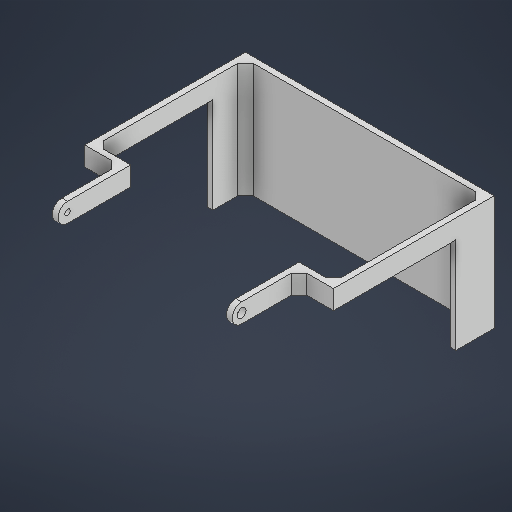
# Autodesk Inventor part: Arm
Saved by Autodesk Inventor 2026.1 (Build 301233020, 233B)
## iProperties
Created: 2025-10-17
Part Number: Arm
Material: Generic
Document SubType Name: Modeling
Designer: Garfieldcmix
Density: 1 g/cm^3
Appearance: Default
Author: Garfieldcmix
Autodesk Inventor part; units mm, degrees
ref_plane "YZ Plane" through (0, 0, 0) normal (1, 0, 0) x (0, 1, 0)
ref_plane "XZ Plane" through (0, 0, 0) normal (0, 1, 0) x (-1, 0, 0)
ref_plane "XY Plane" through (0, 0, 0) normal (0, 0, 1) x (1, 0, 0)
sketch "Sketch1" plane through (0, 0, 0) normal (0, 1, 0) x (-1, 0, 0)
  line L0 (-47, 0) -> (-47, -35)
  line L1 (-47, -35) -> (-65, -35)
  line L2 (-65, -35) -> (-65, -119)
  line L3 (-65, -119) -> (65, -119)
  line L4 (65, -119) -> (65, -35)
  line L5 (65, -35) -> (47, -35)
  line L6 (47, -35) -> (47, 0)
  line L7 (47, 0) -> (44, 0)
  line L8 (44, 0) -> (44, -38)
  line L9 (44, -38) -> (62, -38)
  line L10 (62, -38) -> (62, -116)
  line L11 (62, -116) -> (-62, -116)
  line L12 (-62, -116) -> (-62, -38)
  line L13 (-62, -38) -> (-44, -38)
  line L14 (-44, -38) -> (-44, 0)
  line L15 (-44, 0) -> (-47, 0)
  line L16 (0, -142.8) -> (0, 23.8) construction
  line L17 (91, 0) -> (-91, 0) construction
  dimension "d4" = 3
  dimension "d5" = 3
  dimension "d6" = 3
  dimension "d7" = 3
  dimension "d8" = 35
  dimension "d9" = 130
  dimension "d10" = 84
  dimension "d11" = 88
  constraints: 32 end point, 14 perpendicular, 8 symmetric about line, 2 point on line, 1 horizontal, 1 vertical
  measures "d4" distance of L14.end L0.start
  measures "d5" distance between parallel lines of L13 L1
  measures "d6" distance between parallel lines of L3 L11
  measures "d7" distance between parallel lines of L2 L12
  measures "d8" distance of L0.start L0.end
  measures "d9" distance of L2.end L3.end
  measures "d10" distance of L1.end L2.end
  measures "d11" distance between parallel lines of L14 L8
extrude "Extrusion1" add sketch "Sketch1" along normal blind 10
sketch "Sketch2" plane through (47, 0, 0) normal (1, 0, 0) x (0, 0, -1)
  circle A0 centre (5, 5) radius 2.3
  point P0 (0, 0)
  dimension "d14" = 4.6
  dimension "d15" = 5
  dimension "d16" = 5
  constraints: 1 centre point
  measures "d14" diameter of A0
  measures "d15" horizontal distance of A0.centre point (0, 0)
  measures "d16" horizontal distance of point (0, 0) A0.centre
extrude "Extrusion2" cut sketch "Sketch2" against normal up to surface (3 mm away)
sketch "Sketch3" plane through (-47, 0, -35) normal (-1, 0, 0) x (0, 0, 1)
  circle A0 centre (30, 5) radius 2.3 construction
  circle A1 centre (30, 5) radius 1.5
  point P0 (35, 0)
  dimension "d19" = 3
  constraints: 1 centre point, 1 coincident
  measures "d19" diameter of A1
extrude "Extrusion3" cut sketch "Sketch3" against normal up to surface (3 mm away)
chamfer "Chamfer1" distance 4 angle 45 2 edges at (47, 5, -35) (-47, 5, -35)
chamfer "Chamfer2" distance 4 angle 45 4 edges at (-62, 5, -38) (62, 5, -38) (-62, 5, -116) (62, 5, -116)
fillet "Fillet1" radius 5 4 edges at (45.5, 0, 0) (45.5, 10, 0) (-45.5, 0, 0) (-45.5, 10, 0)
sketch "Sketch4" plane through (0, 0, 0) normal (0, -1, 0) x (1, 0, 0)
  line L0 (62, -112) -> (62, -42) projected
  line L1 (65, -35) -> (65, -119) projected
  line L2 (65, -119) -> (-65, -119) projected
  line L3 (-65, -119) -> (-65, -35) projected
  line L4 (-62, -42) -> (-62, -112) projected
  line L5 (-62, -112) -> (-58, -116) projected
  line L6 (-58, -116) -> (58, -116) projected
  line L7 (58, -116) -> (62, -112) projected
  line L8 (65, -99) -> (62, -99)
  line L9 (-62, -99) -> (-65, -99)
  point P0 (0, 0)
  dimension "d29" = 20
  dimension "d30" = 20
  constraints: 4 end point, 4 point on line, 2 perpendicular
  measures "d29" distance between parallel lines of L2 L9
  measures "d30" distance between parallel lines of L2 L8
extrude "Extrusion4" add sketch "Sketch4" along normal blind 50
body "Solid1"
